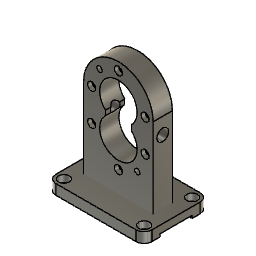
P11 (Autodesk Fusion 360 design; units mm, degrees)
Autodesk Fusion 360 part; units mm, degrees
sketch "Sketch1" plane through (0, 0, 0) normal (0, 0, 1) x (1, 0, 0)
  line L0 (-75, 60) -> (75, 60)
  line L1 (90, 45) -> (90, -45)
  line L2 (75, -60) -> (-75, -60)
  line L3 (-90, -45) -> (-90, 45)
  line L4 (90, 0) -> (-90, 0) construction
  arc A0 (-75, 60) -> (-90, 45) centre (-75, 45) ccw
  arc A1 (90, 45) -> (75, 60) centre (75, 45) ccw
  arc A2 (75, -60) -> (90, -45) centre (75, -45) ccw
  arc A3 (-90, -45) -> (-75, -60) centre (-75, -45) ccw
  line L5 (0, -60) -> (0, 60) construction
  circle A4 centre (-75, 45) radius 7.5
  circle A5 centre (-75, -45) radius 7.5
  circle A6 centre (75, 45) radius 7.5
  circle A7 centre (75, -45) radius 7.5
  point P0 (-90, 60)
  point P1 (90, 60)
  point P2 (-90, -60)
  dimension "d1" = 180
  dimension "d2" = 120
  dimension "d5" = 15
  dimension "d6" = 15
  dimension "d7" = 15
  dimension "d8" = 15
  dimension "d9" = 60
  dimension "d10" = 15
  dimension "d11" = 15
  dimension "d12" = 15
  dimension "d13" = 15
  constraint horizontal L0
  constraint vertical L1
  constraint horizontal L2
  constraint vertical L3
  constraint coincident L3 L4.end
  constraint coincident P0 L3
  constraint coincident P0 L0
  constraint tangent L3 A0
  constraint tangent L0 A0
  constraint coincident L1 L4.start
  constraint coincident P1 L0
  constraint coincident P1 L1
  constraint tangent L0 A1
  constraint tangent L1 A1
  constraint tangent L2 A2
  constraint tangent L1 A2
  constraint coincident P2 L2
  constraint coincident P2 L3
  constraint tangent L2 A3
  constraint tangent L3 A3
  constraint midpoint L2 L5.start
  constraint midpoint L0 L5.end
  constraint coincident origin L5
  constraint coincident origin L4
  constraint concentric A0 A4
  constraint concentric A3 A5
  constraint concentric A1 A6
  constraint concentric A2 A7
  measures "d1" distance of P0 P1
  measures "d2" distance of P0 P2
  measures "d5" radius of A0
  measures "d6" radius of A1
  measures "d7" radius of A2
  measures "d8" radius of A3
  measures "d9" distance of L0 L4
  measures "d10" diameter of A4
  measures "d11" diameter of A5
  measures "d12" diameter of A6
  measures "d13" diameter of A7
extrude "Extrude1" add sketch "Sketch1" along normal blind 19 makes body 1
sketch "Sketch2" plane through (0, 0, 19) normal (0, 0, 1) x (-1, 0, 0)
  circle A0 centre (75, 45) radius 7.5
  circle A1 centre (-75, -45) radius 7.5
  circle A2 centre (-75, 45) radius 7.5
  circle A3 centre (75, -45) radius 7.5
  arc A4 (75, -60) -> (90, -45) centre (75, -45) ccw
  line L0 (90, -45) -> (90, 45)
  arc A5 (90, 45) -> (75, 60) centre (75, 45) ccw
  line L1 (75, 60) -> (-75, 60)
  arc A6 (-75, 60) -> (-90, 45) centre (-75, 45) ccw
  line L2 (-90, 45) -> (-90, -45)
  arc A7 (-90, -45) -> (-75, -60) centre (-75, -45) ccw
  line L3 (-75, -60) -> (75, -60)
  circle A8 centre (75, -45) radius 10
  circle A9 centre (75, 45) radius 10
  circle A10 centre (-75, -45) radius 10
  circle A11 centre (-75, 45) radius 10
  dimension "d16" = 20
  dimension "d17" = 20
  dimension "d18" = 20
  dimension "d19" = 20
  constraint concentric A3 A8
  constraint concentric A0 A9
  constraint concentric A1 A10
  constraint concentric A2 A11
  measures "d16" diameter of A8
  measures "d17" diameter of A9
  measures "d18" diameter of A10
  measures "d19" diameter of A11
extrude "Extrude2" cut sketch "Sketch2" against normal blind 13 contours A8 | A9 | A10 | A11 bodies 1
sketch "Sketch3" plane through (-90, 0, 0) normal (-1, 0, 0) x (0, -1, 0)
  line L0 (-45, 0) -> (45, 0)
  line L1 (45, 0) -> (45, 19)
  line L2 (45, 19) -> (-45, 19)
  line L3 (-45, 19) -> (-45, 0)
  line L4 (30, 5) -> (-30, 5)
  line L5 (-30, 5) -> (-30, -5)
  line L6 (-30, -5) -> (30, -5)
  line L7 (30, -5) -> (30, 5)
  line L8 (30, 5) -> (-30, -5) construction
  line L9 (-30, 5) -> (30, -5) construction
  dimension "d28" = 60
  dimension "d29" = 10
  constraint horizontal L4
  constraint perpendicular L4 L5
  constraint parallel L4 L6
  constraint parallel L5 L7
  constraint coincident L8 origin
  constraint coincident L9 origin
  measures "d28" distance of L5.end L6.end
  measures "d29" distance of L4.end L5.end
extrude "Extrude3" cut sketch "Sketch3" against normal blind 1000 contours L0 L4 L5 L7 bodies 1
sketch "Sketch4" plane through (0, 0, 0) normal (0, 1, 0) x (1, 0, 0)
  line L0 (0, 0) -> (-65, 0)
  line L1 (-65, 0) -> (-65, -168)
  line L2 (-65, -168) -> (0, -168) construction
  line L3 (0, -168) -> (65, -168) construction
  line L4 (65, 0) -> (0, 0)
  line L5 (65, -168) -> (65, 0)
  arc A0 (-65, -168) -> (65, -168) centre (0, -168) ccw
  line L6 (0, -168) -> (0, -108) construction
  line L7 (0, -108) -> (0, -138)
  line L8 (0, -138) -> (24, -138) construction
  line L9 (0, -138) -> (-24, -138) construction
  line L10 (24, -138) -> (24, -142.5245)
  line L11 (24, -138) -> (24, -133.4755)
  line L12 (-24, -138) -> (-24, -137)
  line L13 (-24, -137) -> (-24, -133.4755)
  line L14 (-24, -138) -> (-24, -142.5245)
  arc A1 (24, -133.4755) -> (-24, -133.4755) centre (0, -108) ccw
  arc A2 (-24, -142.5245) -> (24, -142.5245) centre (0, -168) ccw
  line L15 (65, -142.5245) -> (-65, -142.5245) construction
  arc A3 (-43.0232, -142.5245) -> (43.0232, -142.5245) centre (0, -168) ccw construction
  line L16 (65, -133.4755) -> (-65, -133.4755) construction
  arc A4 (43.0232, -133.4755) -> (-43.0232, -133.4755) centre (0, -108) ccw construction
  circle A5 centre (50, -168) radius 6
  circle A6 centre (0, -218) radius 6
  circle A7 centre (-50, -168) radius 6
  circle A8 centre (-50, -108) radius 6
  circle A9 centre (0, -58) radius 6
  circle A10 centre (50, -108) radius 6
  line L17 (0, -168) -> (-35.3553, -203.3553)
  line L18 (0, -168) -> (-50, -168) construction
  circle A11 centre (-35.3553, -203.3553) radius 5
  circle A12 centre (35.3553, -72.6447) radius 5
  line L19 (0, -108) -> (35.3553, -72.6447)
  line L20 (0, -108) -> (50, -108) construction
  dimension "d32" = 65
  dimension "d34" = 130
  dimension "d35" = 168
  dimension "d37" = 168
  dimension "d38" = 60
  dimension "d39" = 70
  dimension "d40" = 70
  dimension "d41" = 24
  dimension "d42" = 24
  dimension "d46" = 12
  dimension "d48" = -180
  dimension "d49" = 50
  dimension "d51" = 45
  dimension "d52" = 50
  dimension "d53" = 10
  dimension "d54" = 45
  dimension "d55" = 10
  dimension "d56" = 50
  constraint coincident L0.start L4.end
  constraint horizontal L0
  constraint perpendicular L0 L1
  constraint perpendicular L1 L2
  constraint coincident L2.end L3.start
  constraint parallel L2 L3
  constraint tangent L5 A0
  constraint perpendicular L2 L6
  constraint coincident L6.end L7.start
  constraint concentric A0 A2
  constraint midpoint L6 L7.end
  constraint perpendicular L6 L8
  constraint perpendicular L6 L9
  constraint perpendicular L8 L10
  constraint perpendicular L8 L11
  constraint perpendicular L9 L12
  constraint perpendicular L9 L13
  constraint perpendicular L9 L14
  constraint coincident L5 L15.start
  constraint coincident L1 L15.end
  constraint perpendicular L1 L15
  constraint coincident L15 A3.end
  constraint coincident L15 A3.start
  constraint coincident L5 L16.start
  constraint coincident L1 L16.end
  constraint perpendicular L1 L16
  constraint coincident L16 A4.start
  constraint coincident L16 A4.end
  constraint coincident L3 A5.centre
  constraint coincident A3 A5.centre
  constraint symmetric L9 A5 A10
  constraint symmetric L9 A6 A9
  constraint symmetric L9 A7 A8
  constraint horizontal L18
  constraint coincident L17.end A11.centre
  constraint horizontal L20
  constraint coincident A4 A12.centre
  constraint coincident A12.centre L19.end
  measures "d32" distance of L0.start L0.end
  measures "d34" diameter of A0
  measures "d35" distance of L0.start L2.end
  measures "d37" distance of L3.end L4.start
  measures "d38" distance of L2.end L6.end
  measures "d39" diameter of A1
  measures "d40" diameter of A2
  measures "d41" distance of L7.end L8.end
  measures "d42" distance of L7.end L9.end
  measures "d46" diameter of A5
  measures "d49" distance of L2.end A5.centre
  measures "d51" angle of L17 L18
  measures "d52" distance of L2.end L17.end
  measures "d53" diameter of A11
  measures "d54" angle of L19 L20
  measures "d55" diameter of A12
  measures "d56" distance of L6.end A12.centre
extrude "Extrude4" add sketch "Sketch4" along normal mid plane 36 separate body makes body 2
sketch "Sketch5" plane through (0, 18, 0) normal (0, 1, 0) x (-1, 0, 0)
  circle A0 centre (35.3553, 203.3553) radius 5
  circle A1 centre (-50, 168) radius 6
  line L0 (24, 142.5245) -> (24, 133.4755)
  arc A2 (-24, 133.4755) -> (24, 133.4755) centre (0, 108) ccw
  line L1 (-24, 133.4755) -> (-24, 142.5245)
  arc A3 (24, 142.5245) -> (-24, 142.5245) centre (0, 168) ccw
  circle A4 centre (50, 108) radius 6
  circle A5 centre (-50, 108) radius 6
  circle A6 centre (0, 58) radius 6
  circle A7 centre (0, 218) radius 6
  circle A8 centre (50, 168) radius 6
  circle A9 centre (-35.3553, 72.6447) radius 5
  arc A10 (65, 168) -> (-65, 168) centre (0, 168) ccw
  line L2 (-65, 168) -> (-65, 0)
  line L3 (-65, 0) -> (65, 0)
  line L4 (65, 0) -> (65, 168)
  circle A11 centre (-50, 108) radius 7.5
  circle A12 centre (50, 108) radius 7.5
  circle A13 centre (0, 58) radius 7.5
  circle A14 centre (50, 168) radius 7.5
  circle A15 centre (-50, 168) radius 7.5
  circle A16 centre (0, 218) radius 7.5
  dimension "d59" = 15
  dimension "d60" = 15
  dimension "d61" = 15
  dimension "d62" = 15
  dimension "d63" = 15
  dimension "d64" = 15
  constraint concentric A5 A11
  constraint concentric A4 A12
  constraint concentric A6 A13
  constraint concentric A8 A14
  constraint concentric A1 A15
  constraint concentric A7 A16
  measures "d59" diameter of A11
  measures "d60" diameter of A12
  measures "d61" diameter of A13
  measures "d62" diameter of A14
  measures "d63" diameter of A15
  measures "d64" diameter of A16
extrude "Extrude5" cut sketch "Sketch5" against normal blind 8 contours A8 | A11 | A12 | A13 | A15 | A16 bodies 2
sketch "Sketch6" plane through (0, -18, 0) normal (0, -1, 0) x (1, 0, 0)
  circle A0 centre (-35.3553, 203.3553) radius 5
  circle A1 centre (50, 168) radius 6
  line L0 (-24, 133.4755) -> (-24, 142.5245)
  arc A2 (24, 142.5245) -> (-24, 142.5245) centre (0, 168) ccw
  line L1 (24, 142.5245) -> (24, 133.4755)
  arc A3 (-24, 133.4755) -> (24, 133.4755) centre (0, 108) ccw
  circle A4 centre (-50, 108) radius 6
  circle A5 centre (50, 108) radius 6
  circle A6 centre (0, 58) radius 6
  circle A7 centre (0, 218) radius 6
  circle A8 centre (-50, 168) radius 6
  circle A9 centre (35.3553, 72.6447) radius 5
  arc A10 (65, 168) -> (-65, 168) centre (0, 168) ccw
  line L2 (-65, 168) -> (-65, 0)
  line L3 (-65, 0) -> (65, 0)
  line L4 (65, 0) -> (65, 168)
  circle A11 centre (0, 58) radius 7.5
  circle A12 centre (50, 108) radius 7.5
  circle A13 centre (-50, 108) radius 7.5
  circle A14 centre (-50, 168) radius 7.5
  circle A15 centre (50, 168) radius 7.5
  circle A16 centre (0, 218) radius 7.5
  dimension "d67" = 15
  dimension "d68" = 15
  dimension "d69" = 15
  dimension "d70" = 15
  dimension "d71" = 15
  dimension "d72" = 15
  constraint concentric A6 A11
  constraint concentric A5 A12
  constraint concentric A4 A13
  constraint concentric A8 A14
  constraint concentric A1 A15
  constraint concentric A7 A16
  measures "d67" diameter of A11
  measures "d68" diameter of A12
  measures "d69" diameter of A13
  measures "d70" diameter of A14
  measures "d71" diameter of A15
  measures "d72" diameter of A16
extrude "Extrude6" cut sketch "Sketch6" against normal blind 8 contours A11 | A12 | A13 | A14 | A15 | A16 bodies 2
sketch "Sketch7" plane through (-65, 0, 0) normal (-1, 0, 0) x (0, -1, 0)
  line L0 (18, 168) -> (-18, 168)
  line L1 (-18, 168) -> (-18, 0)
  line L2 (-18, 0) -> (18, 0)
  line L3 (18, 0) -> (18, 168)
  line L4 (18, 0) -> (18, 138) construction
  line L5 (18, 138) -> (-18, 138) construction
  circle A0 centre (0, 138) radius 9
  dimension "d75" = 138
  dimension "d76" = 18
  constraint coincident L2.end L3.start
  constraint perpendicular L2 L4
  constraint coincident L1 L5.end
  constraint perpendicular L1 L5
  constraint midpoint L5 A0.centre
  measures "d75" distance of L2.end L4.end
  measures "d76" diameter of A0
extrude "Extrude7" cut sketch "Sketch7" against normal blind 160 contours A0 bodies 2
sketch "Sketch8" plane through (-65, 0, 0) normal (-1, 0, 0) x (0, -1, 0)
  circle A0 centre (0, 138) radius 9
  line L0 (18, 168) -> (-18, 168)
  line L1 (-18, 168) -> (-18, 0)
  line L2 (-18, 0) -> (18, 0)
  line L3 (18, 0) -> (18, 168)
  circle A1 centre (0, 138) radius 11
  dimension "d79" = 22
  constraint concentric A0 A1
  measures "d79" diameter of A1
extrude "Extrude8" cut sketch "Sketch8" against normal blind 15 contours A1 bodies 2
sketch "Sketch9" plane through (65, 0, 0) normal (1, 0, 0) x (0, 1, 0)
  circle A0 centre (0, 138) radius 9
  line L0 (-18, 0) -> (18, 0)
  line L1 (18, 0) -> (18, 168)
  line L2 (18, 168) -> (-18, 168)
  line L3 (-18, 168) -> (-18, 0)
  circle A1 centre (0, 138) radius 11
  dimension "d82" = 22
  constraint concentric A0 A1
  measures "d82" diameter of A1
extrude "Extrude9" cut sketch "Sketch9" against normal blind 15 contours A1 bodies 2
extrude "Extrude10" cut sketch "Sketch3" against normal blind 200 contours L0 L4 L5 L7 bodies 2
